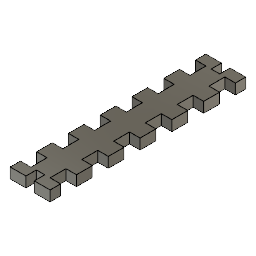
retroside (Autodesk Fusion 360 design; units mm, degrees)
Autodesk Fusion 360 part; units mm, degrees
sketch "Sketch1" plane through (0, 0, 0) normal (0, 0, 1) x (1, 0, 0)
  line L0 (0, 0) -> (9, 0)
  line L1 (9, 0) -> (9, 83)
  line L2 (9, 83) -> (0, 83)
  line L3 (0, 83) -> (0, 0)
  dimension "d5" = 9
  dimension "d6" = 83
  constraint horizontal L0
  constraint vertical L1
  constraint horizontal L2
  constraint vertical L3
  constraint coincident L0.start L3.end
  measures "d5" distance of L0.start L0.end
  measures "d6" distance of L0.start L2.end
extrude "Extrude1" add sketch "Sketch1" along normal blind 5
sketch "Sketch2" plane through (9, 0, 0) normal (1, 0, 0) x (0, 1, 0)
  line L0 (0, 0) -> (83, 0)
  line L1 (83, 0) -> (83, 5)
  line L2 (83, 5) -> (0, 5)
  line L3 (0, 5) -> (0, 0)
  line L4 (7.5455, 5) -> (15.0909, 5)
  line L5 (15.0909, 5) -> (15.0909, 0)
  line L6 (15.0909, 0) -> (7.5455, 0)
  line L7 (7.5455, 0) -> (7.5455, 5)
  line L8 (22.6364, 0) -> (22.6364, 5)
  line L9 (22.6364, 5) -> (30.1818, 5)
  line L10 (30.1818, 0) -> (22.6364, 0)
  line L11 (30.1818, 5) -> (30.1818, 0)
  line L12 (37.7273, 0) -> (37.7273, 5)
  line L13 (37.7273, 5) -> (45.2727, 5)
  line L14 (45.2727, 0) -> (37.7273, 0)
  line L15 (45.2727, 5) -> (45.2727, 0)
  line L16 (52.8182, 0) -> (52.8182, 5)
  line L17 (52.8182, 5) -> (60.3636, 5)
  line L18 (60.3636, 0) -> (52.8182, 0)
  line L19 (60.3636, 5) -> (60.3636, 0)
  line L20 (67.9091, 0) -> (67.9091, 5)
  line L21 (67.9091, 5) -> (75.4545, 5)
  line L22 (75.4545, 0) -> (67.9091, 0)
  line L23 (75.4545, 5) -> (75.4545, 0)
  dimension "d9" = 7.5455
  dimension "d10" = 7.5455
  dimension "d13" = 60.3636
  dimension "d14" = 0
  constraint horizontal L4
  constraint vertical L5
  constraint horizontal L6
  constraint vertical L7
  constraint coincident L0 L5.end
  constraint coincident L2 L4.start
  measures "d9" distance of L4.start L4.end
  measures "d10" distance of L0.start L6.end
extrude "Extrude2" add sketch "Sketch2" along normal blind 5 contours L0 L2 L4 L5 L6 L7 | L0 L2 L8 L9 L10 L11 | L0 L2 L12 L13 L14 L15 | L0 L2 L16 L17 L18 L19 | L0 L2 L20 L21 L22 L23
sketch "Sketch3" plane through (0, 0, 0) normal (-1, 0, 0) x (0, -1, 0)
  line L0 (-83, 0) -> (0, 0)
  line L1 (0, 0) -> (0, 5)
  line L2 (0, 5) -> (-83, 5)
  line L3 (-83, 5) -> (-83, 0)
  line L4 (-75.4545, 5) -> (-67.9091, 5)
  line L5 (-67.9091, 5) -> (-67.9091, 0)
  line L6 (-67.9091, 0) -> (-75.4545, 0)
  line L7 (-75.4545, 0) -> (-75.4545, 5)
  line L8 (-60.3636, 0) -> (-60.3636, 5)
  line L9 (-60.3636, 5) -> (-52.8182, 5)
  line L10 (-52.8182, 0) -> (-60.3636, 0)
  line L11 (-52.8182, 5) -> (-52.8182, 0)
  line L12 (-45.2727, 0) -> (-45.2727, 5)
  line L13 (-45.2727, 5) -> (-37.7273, 5)
  line L14 (-37.7273, 0) -> (-45.2727, 0)
  line L15 (-37.7273, 5) -> (-37.7273, 0)
  line L16 (-30.1818, 0) -> (-30.1818, 5)
  line L17 (-30.1818, 5) -> (-22.6364, 5)
  line L18 (-22.6364, 0) -> (-30.1818, 0)
  line L19 (-22.6364, 5) -> (-22.6364, 0)
  line L20 (-15.0909, 0) -> (-15.0909, 5)
  line L21 (-15.0909, 5) -> (-7.5455, 5)
  line L22 (-7.5455, 0) -> (-15.0909, 0)
  line L23 (-7.5455, 5) -> (-7.5455, 0)
  point P0 (-75.4545, 5)
  dimension "d17" = 7.5455
  dimension "d20" = 60.3636
  dimension "d21" = 0
  constraint horizontal L4
  constraint vertical L5
  constraint horizontal L6
  constraint vertical L7
  constraint coincident L0 L5.end
  constraint coincident P0 L4.start
  measures "d17" distance of P0 L4.end
extrude "Extrude3" add sketch "Sketch3" along normal blind 5 contours L0 L2 L4 L5 L6 L7 | L0 L2 L8 L9 L10 L11 | L0 L2 L12 L13 L14 L15 | L0 L2 L16 L17 L18 L19 | L0 L2 L20 L21 L22 L23
sketch "Sketch4" plane through (0, 0, 0) normal (0, -1, 0) x (1, 0, 0)
  line L0 (0, 0) -> (9, 0)
  line L1 (9, 0) -> (9, 5)
  line L2 (9, 5) -> (0, 5)
  line L3 (0, 5) -> (0, 0)
sketch "Sketch5" plane through (0, 0, 0) normal (0, 0, 1) x (1, 0, 0)
  line L0 (-5, 0) -> (14, 0)
  line L1 (14, 0) -> (14, -5)
  line L2 (14, -5) -> (-5, -5)
  line L3 (-5, -5) -> (-5, 0)
  line L4 (0, 7.5455) -> (0, 0) construction
  line L5 (0, 0) -> (9, 0)
  point P0 (-5, 7.5455)
  dimension "d24" = 5
  dimension "d25" = 19
  dimension "d44" = 5
  constraint horizontal L0
  constraint vertical L1
  constraint horizontal L2
  constraint vertical L3
  constraint collinear L0 L5
  measures "d24" distance of L0.end L1.end
  measures "d25" distance of L1.end L2.end
  measures "d44" distance of L0.end L5.end
extrude "Extrude4" cut sketch "Sketch5" along normal blind 5
extrude "Extrude5" add sketch "Sketch5" along normal blind 5
sketch "Sketch6" plane through (0, 0, 0) normal (0, 0, 1) x (1, 0, 0)
  line L0 (-5, 83) -> (14, 83)
  line L1 (14, 83) -> (14, 88)
  line L2 (14, 88) -> (-5, 88)
  line L3 (-5, 88) -> (-5, 83)
  line L4 (9, 83) -> (0, 83)
  point P0 (0, 83)
  point P1 (-5, 75.4545)
  dimension "d31" = 19
  dimension "d32" = 5
  dimension "d43" = 5
  constraint horizontal L0
  constraint vertical L1
  constraint horizontal L2
  constraint vertical L3
  constraint collinear L0 L4
  measures "d31" distance of L0.start L0.end
  measures "d32" distance of L0.start L2.end
  measures "d43" distance of L0.start P0
extrude "Extrude6" cut sketch "Sketch6" along normal blind 5
extrude "Extrude7" add sketch "Sketch6" along normal blind 5
sketch "Sketch7" plane through (0, 0, 5) normal (0, 0, 1) x (-1, 0, 0)
  line L0 (0, -83) -> (0, -75.4545)
  line L1 (0, -75.4545) -> (5, -75.4545)
  line L2 (5, -75.4545) -> (5, -67.9091)
  line L3 (5, -67.9091) -> (0, -67.9091)
  line L4 (0, -67.9091) -> (0, -60.3636)
  line L5 (0, -60.3636) -> (5, -60.3636)
  line L6 (5, -60.3636) -> (5, -52.8182)
  line L7 (5, -52.8182) -> (0, -52.8182)
  line L8 (0, -52.8182) -> (0, -45.2727)
  line L9 (0, -45.2727) -> (5, -45.2727)
  line L10 (5, -45.2727) -> (5, -37.7273)
  line L11 (5, -37.7273) -> (0, -37.7273)
  line L12 (0, -37.7273) -> (0, -30.1818)
  line L13 (0, -30.1818) -> (5, -30.1818)
  line L14 (5, -30.1818) -> (5, -22.6364)
  line L15 (5, -22.6364) -> (0, -22.6364)
  line L16 (0, -22.6364) -> (0, -15.0909)
  line L17 (0, -15.0909) -> (5, -15.0909)
  line L18 (5, -15.0909) -> (5, -7.5455)
  line L19 (5, -7.5455) -> (0, -7.5455)
  line L20 (0, -7.5455) -> (0, 0)
  line L21 (0, 0) -> (5, 0)
  line L22 (5, 0) -> (5, 5)
  line L23 (5, 5) -> (-14, 5)
  line L24 (-14, 5) -> (-14, 0)
  line L25 (-14, 0) -> (-9, 0)
  line L26 (-9, 0) -> (-9, -7.5455)
  line L27 (-9, -7.5455) -> (-14, -7.5455)
  line L28 (-14, -7.5455) -> (-14, -15.0909)
  line L29 (-14, -15.0909) -> (-9, -15.0909)
  line L30 (-9, -15.0909) -> (-9, -22.6364)
  line L31 (-9, -22.6364) -> (-14, -22.6364)
  line L32 (-14, -22.6364) -> (-14, -30.1818)
  line L33 (-14, -30.1818) -> (-9, -30.1818)
  line L34 (-9, -30.1818) -> (-9, -37.7273)
  line L35 (-9, -37.7273) -> (-14, -37.7273)
  line L36 (-14, -37.7273) -> (-14, -45.2727)
  line L37 (-14, -45.2727) -> (-9, -45.2727)
  line L38 (-9, -45.2727) -> (-9, -52.8182)
  line L39 (-9, -52.8182) -> (-14, -52.8182)
  line L40 (-14, -52.8182) -> (-14, -60.3636)
  line L41 (-14, -60.3636) -> (-9, -60.3636)
  line L42 (-9, -60.3636) -> (-9, -67.9091)
  line L43 (-9, -67.9091) -> (-14, -67.9091)
  line L44 (-14, -67.9091) -> (-14, -75.4545)
  line L45 (-14, -75.4545) -> (-9, -75.4545)
  line L46 (-9, -75.4545) -> (-9, -83)
  line L47 (-9, -83) -> (-14, -83)
  line L48 (-14, -83) -> (-14, -88)
  line L49 (-14, -88) -> (5, -88)
  line L50 (5, -88) -> (5, -83)
  line L51 (5, -83) -> (0, -83)
  line L52 (-2.5, 0) -> (-6.5, 0)
  line L53 (-6.5, 0) -> (-6.5, 5)
  line L54 (-6.5, 5) -> (-2.5, 5)
  line L55 (-2.5, 5) -> (-2.5, 0)
  line L56 (-6.5, 0) -> (-9, 0) construction
  line L57 (0, 0) -> (-2.5, 0) construction
  line L58 (-2.5, -88) -> (-6.5, -88)
  line L59 (-6.5, -88) -> (-6.5, -83)
  line L60 (-6.5, -83) -> (-2.5, -83)
  line L61 (-2.5, -83) -> (-2.5, -88)
  line L62 (-6.5, -83) -> (-9, -83) construction
  line L63 (-2.5, -83) -> (0, -83) construction
  dimension "d41" = 4
  dimension "d42" = 5
  dimension "d45" = 5
  dimension "d46" = 4
  constraint horizontal L52
  constraint vertical L53
  constraint horizontal L54
  constraint vertical L55
  constraint coincident L23 L53.end
  constraint coincident L25.end L26.start
  constraint coincident L20.end L21.start
  constraint equal L56 L57
  constraint horizontal L58
  constraint vertical L59
  constraint horizontal L60
  constraint vertical L61
  constraint coincident L49 L58.start
  constraint coincident L46.end L47.start
  constraint coincident L0.start L51.end
  constraint equal L62 L63
  measures "d41" distance of L52.start L52.end
  measures "d42" distance of L52.start L54.end
  measures "d45" distance of L58.start L60.end
  measures "d46" distance of L59.end L60.end
extrude "Extrude9" cut sketch "Sketch7" against normal blind 5 contours L23 L52 L53 L54 L55
extrude "Extrude8" cut sketch "Sketch7" against normal blind 5 contours L49 L58 L59 L60 L61
equation "paksus = 5 mm"
equation "pikkus = 83 mm"
equation "pikkus_tapp = pikkus / 11"
equation "laius = 9 mm"
equation "d5 = laius"
equation "d6 = pikkus"
equation "d7 = paksus"
equation "d9 = pikkus_tapp"
equation "d10 = pikkus_tapp"
equation "d13 = pikkus - 2 * pikkus_tapp - pikkus_tapp"
equation "d15 = paksus"
equation "d17 = pikkus_tapp"
equation "d20 = pikkus - 2 * pikkus_tapp - pikkus_tapp"
equation "d22 = paksus"
equation "d24 = paksus"
equation "d25 = 2 * paksus + laius"
equation "d27 = paksus"
equation "d29 = paksus"
equation "d31 = 2 * paksus + laius"
equation "d32 = paksus"
equation "d34 = paksus"
equation "d36 = paksus"
equation "d44 = paksus"
equation "d45 = paksus"
equation "d47 = -paksus"
equation "d49 = -paksus"
